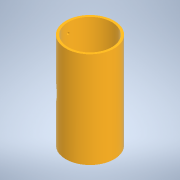
# Autodesk Inventor part: Tubo Interior
Saved by Autodesk Inventor 2020.3 (Build 243373000, 373)
## iProperties
Created: 2020-07-25
Part Number: Tubo Interior
Material: PVC-Piping
Document SubType Name: Modeling
Designer: juanp
Density: 1.4 g/cm^3
Appearance: Smooth - White
Author: juanp
Autodesk Inventor part; units mm, degrees
ref_plane "YZ Plane" through (0, 0, 0) normal (1, 0, 0) x (0, 1, 0)
ref_plane "XZ Plane" through (0, 0, 0) normal (0, 1, 0) x (-1, 0, 0)
ref_plane "XY Plane" through (0, 0, 0) normal (0, 0, 1) x (1, 0, 0)
sketch "Sketch2" plane through (0, 0, 0) normal (0, 1, 0) x (-1, 0, 0)
  circle A0 centre (0, 0) radius 30.16
  circle A1 centre (0, 0) radius 27.24
  dimension "d0" = 60.32
  dimension "d1" = 54.48
  constraints: 2 centre point, 2 coincident
  measures "d0" diameter of A0
  measures "d1" diameter of A1
extrude "Extrusion1" add sketch "Sketch2" along normal blind 120
sketch "Sketch3" plane through (0, 0, 0) normal (1, 0, 0) x (0, 1, 0)
  line L0 (0, -30.16) -> (0, 30.16) projected
  line L1 (120, -30.16) -> (120, 30.16) projected
  line L2 (0, -30.16) -> (120, 30.16) construction
  line L3 (120, -30.16) -> (0, 30.16) construction
  circle A0 centre (60, 0) radius 25.4
  line L4 (120, 27.24) -> (0, 27.24) projected
  line L5 (120, 0) -> (102.125, 0)
  line L6 (0, 0) -> (17.875, 0)
  circle A1 centre (17.875, 0) radius 2.55
  circle A2 centre (102.125, 0) radius 2.55
  dimension "d6" = 50.8
  dimension "d7" = 17.875
  dimension "d8" = 17.875
  dimension "d9" = 5.1
  dimension "d10" = 5.1
  constraints: 8 end point, 3 centre point, 2 coincident, 2 horizontal, 2 midpoint
  measures "d6" diameter of A0
  measures "d7" distance of L5.start L5.end
  measures "d8" distance of L6.start L6.end
  measures "d9" diameter of A1
  measures "d10" diameter of A2
extrude "Extrusion2" cut sketch "Sketch3" against normal up to next
body "Solid1"
